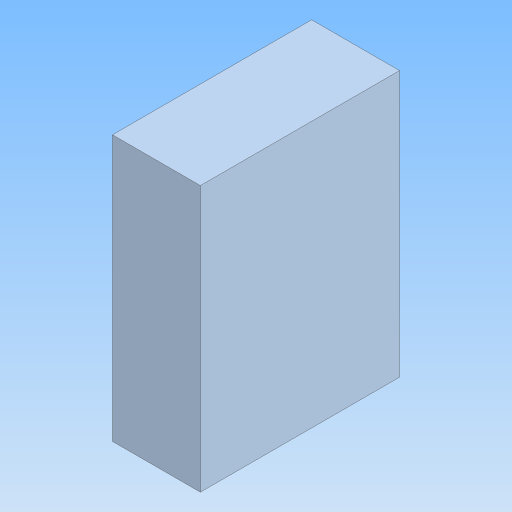
# Autodesk Inventor part: Wellennut
Saved by Autodesk Inventor 2024.4 (Build 284460000, 460)
## iProperties
Created: 2026-01-19
Part Number: Wellennut
Material: Generisch
Document SubType Name: Modeling
Designer: windows-desktop
Density: 1 g/cm^3
Appearance: Vorgabe
Mass: 1.9866 g
Surface Area: 10.6354 cm^2
Volume: 1.9866 cm^3
Masse[kg]: 0,002 kg
Autodesk Inventor part; units mm, degrees
ref_plane "YZ Plane" through (0, 0, 0) normal (1, 0, 0) x (0, 1, 0)
ref_plane "XZ Plane" through (0, 0, 0) normal (0, 1, 0) x (-1, 0, 0)
ref_plane "XY Plane" through (0, 0, 0) normal (0, 0, 1) x (1, 0, 0)
sketch "Skizze1" plane through (0, 0, 0) normal (0, 1, 0) x (-1, 0, 0)
  line L0 (3.311, 10) -> (-3.311, 10)
  line L1 (-3.311, 10) -> (-3.311, -10)
  line L2 (-3.311, -10) -> (3.311, -10)
  line L3 (3.311, -10) -> (3.311, 10)
  line L4 (4.6354, 0) -> (-4.6354, 0) construction
  line L5 (0, -14) -> (0, 14) construction
  point P0 (0, 0)
  dimension "d0" = 6.622
  dimension "d1" = 20
  constraints: 8 end point, 2 parallel, 1 horizontal, 1 perpendicular, 2 other
  measures "d0" distance of L2.end L1.end
  measures "d1" distance of L1.end L0.end
extrude "Extrusion1" add sketch "Skizze1" along normal blind 15
